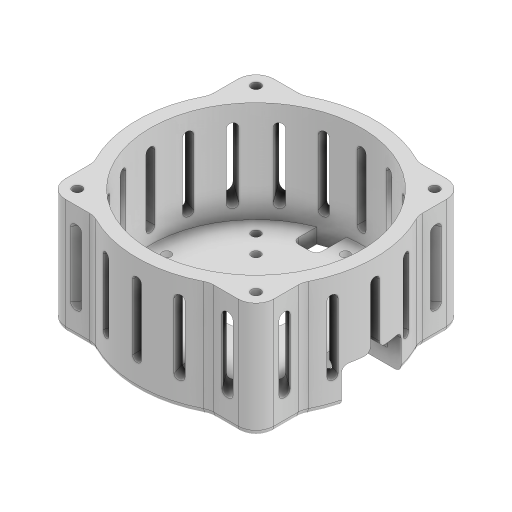
# Autodesk Inventor part: casing
Saved by Autodesk Inventor 2024.3 (Build 283343000, 343)
## iProperties
Created: 2025-08-30
Part Number: casing
Material: Generic
Document SubType Name: Modeling
Designer: danie
Density: 1 g/cm^3
Appearance: Default
Author: danie
Autodesk Inventor part; units mm, degrees
ref_plane "YZ Plane" through (0, 0, 0) normal (1, 0, 0) x (0, 1, 0)
ref_plane "XZ Plane" through (0, 0, 0) normal (0, 1, 0) x (-1, 0, 0)
ref_plane "XY Plane" through (0, 0, 0) normal (0, 0, 1) x (1, 0, 0)
sketch "Sketch1" plane through (0, 0, 0) normal (0, 1, 0) x (-1, 0, 0)
  circle A0 centre (0, 0) radius 34.5
  line L0 (-15, 15) -> (15, 15)
  line L1 (15, 15) -> (15, -15)
  line L2 (15, -15) -> (-15, -15)
  line L3 (-15, -15) -> (-15, 15)
  line L4 (-15, 15) -> (15, -15) construction
  line L5 (15, 15) -> (-15, -15) construction
  circle A1 centre (0, 0) radius 40
  circle A2 centre (0, 0) radius 35.5
  line L6 (-35, 35) -> (35, 35)
  line L7 (35, 35) -> (35, -35)
  line L8 (35, -35) -> (-35, -35)
  line L9 (-35, -35) -> (-35, 35)
  line L10 (-35, 35) -> (35, -35) construction
  line L11 (35, 35) -> (-35, -35) construction
  circle A3 centre (15, 15) radius 1.5
  circle A4 centre (15, -15) radius 1.5
  circle A5 centre (-15, -15) radius 1.5
  circle A6 centre (-15, 15) radius 1.5
  line L12 (21, 21) -> (-21, 21)
  line L13 (-21, 21) -> (-21, -21)
  line L14 (-21, -21) -> (21, -21)
  line L15 (21, -21) -> (21, 21)
  line L16 (21, 21) -> (-21, -21) construction
  line L17 (-21, 21) -> (21, -21) construction
  circle A7 centre (0, 0) radius 10
  circle A8 centre (21, 21) radius 1.5
  circle A9 centre (21, -21) radius 1.5
  circle A10 centre (-21, 21) radius 1.5
  circle A11 centre (-21, -21) radius 1.5
  line L18 (0, 0) -> (30, 0)
  circle A12 centre (30, 0) radius 1.5
  circle A13 centre (0, 30) radius 1.5
  circle A14 centre (-30, 0) radius 1.5
  circle A15 centre (0, -30) radius 1.5
  line L19 (-45.5, 10) -> (-27.5, 10)
  line L20 (-25.5, 8) -> (-25.5, -8)
  line L21 (-27.5, -10) -> (-45.5, -10)
  line L22 (-45.5, -10) -> (-45.5, 10)
  line L23 (-45.5, 10) -> (-25.5, -10) construction
  line L24 (-25.5, 10) -> (-45.5, -10) construction
  arc A16 (-25.5, 8) -> (-27.5, 10) centre (-27.5, 8) ccw
  arc A17 (-27.5, -10) -> (-25.5, -8) centre (-27.5, -8) ccw
  line L25 (0, 35) -> (0, -35)
  line L26 (35, 35) -> (0, 35)
  line L27 (17.5, 35) -> (17.5, -35)
  line L28 (17.5, 35) -> (0, 35)
  line L29 (8.75, 35) -> (8.75, -35)
  line L30 (4.75, 45) -> (12.75, 45)
  line L31 (12.75, 45) -> (12.75, 27)
  line L32 (10.75, 25) -> (6.75, 25)
  line L33 (4.75, 27) -> (4.75, 45)
  line L34 (4.75, 45) -> (12.75, 25) construction
  line L35 (12.75, 45) -> (4.75, 25) construction
  arc A18 (10.75, 25) -> (12.75, 27) centre (10.75, 27) ccw
  arc A19 (4.75, 27) -> (6.75, 25) centre (6.75, 27) ccw
  line L36 (4.75, -45) -> (12.75, -45)
  line L37 (12.75, -45) -> (12.75, -27)
  line L38 (10.75, -25) -> (6.75, -25)
  line L39 (4.75, -27) -> (4.75, -45)
  arc A20 (12.75, -27) -> (10.75, -25) centre (10.75, -27) ccw
  arc A21 (6.75, -25) -> (4.75, -27) centre (6.75, -27) ccw
  line L40 (-4.75, 45) -> (-12.75, 45)
  line L41 (-12.75, 45) -> (-12.75, 27)
  line L42 (-10.75, 25) -> (-6.75, 25)
  line L43 (-4.75, 27) -> (-4.75, 45)
  arc A22 (-12.75, 27) -> (-10.75, 25) centre (-10.75, 27) ccw
  arc A23 (-6.75, 25) -> (-4.75, 27) centre (-6.75, 27) ccw
  line L44 (-12.75, -45) -> (-12.75, -27)
  arc A24 (-10.75, -25) -> (-12.75, -27) centre (-10.75, -27) ccw
  line L45 (-10.75, -25) -> (-6.75, -25)
  arc A25 (-4.75, -27) -> (-6.75, -25) centre (-6.75, -27) ccw
  line L46 (-4.75, -27) -> (-4.75, -45)
  line L47 (-4.75, -45) -> (-12.75, -45)
  point P0 (19.3649, 35)
  point P1 (-19.3649, 35)
  point P2 (-35, 19.3649)
  point P3 (-35, -19.3649)
  point P4 (-19.3649, -35)
  point P5 (19.3649, -35)
  point P6 (35, -19.3649)
  point P7 (35, 19.3649)
  point P8 (-5.9372, -35)
  point P9 (5.9372, -35)
  point P10 (5.9372, 35)
  point P11 (-5.9372, 35)
  point P12 (-35.5, 0)
  point P13 (12.75, 33.1314)
  point P14 (4.75, 35.1808)
  point P15 (-4.75, 35.1808)
  point P16 (-12.75, 33.1314)
  point P17 (-34.0624, 10)
  point P18 (-34.0624, -10)
  point P19 (-12.75, -33.1314)
  point P20 (-4.75, -35.1808)
  point P21 (4.75, -35.1808)
  point P22 (12.75, -33.1314)
  dimension "d30" = 71
  dimension "d0" = 69
  dimension "d1" = 30
  dimension "d2" = 30
  dimension "d3" = 80
  dimension "d4" = 70
  dimension "d5" = 70
  dimension "d6" = 3
  dimension "d7" = 3
  dimension "d8" = 3
  dimension "d9" = 3
  dimension "d10" = 20
  dimension "d11" = 3
  dimension "d12" = 42
  dimension "d15" = 42
  dimension "d18" = 42
  dimension "d25" = 3
  dimension "d28" = 360
  dimension "d31" = 20
  dimension "d32" = 20
  dimension "d33" = 2
  dimension "d34" = 8
  dimension "d35" = 20
  dimension "d36" = 2
  constraints: 96 end point, 25 centre point, 24 symmetric about line, 20 point on circle, 14 midpoint, 11 point on line, 10 coincident, 10 parallel, 8 tangent, 7 horizontal, 7 perpendicular, 2 collinear, 2 equal radius, 1 vertical, 24 other
  measures "d0" diameter of A0
  measures "d1" distance between parallel lines of L2 L0
  measures "d2" distance between parallel lines of L3 L1
  measures "d3" diameter of A1
  measures "d4" distance between parallel lines of L8 L6
  measures "d5" distance between parallel lines of L9 L7
  measures "d6" diameter of A3
  measures "d7" diameter of A4
  measures "d8" diameter of A5
  measures "d9" diameter of A6
  measures "d10" diameter of A7
  measures "d11" diameter of A8
  measures "d12" distance between parallel lines of L14 L12
  measures "d15" distance of A8.centre A9.centre
  measures "d18" distance of A8.centre A10.centre
  measures "d25" diameter of A12
  measures "d31" distance between parallel lines of L21 L19
  measures "d32" distance between parallel lines of L22 L20
  measures "d33" radius of A16
  measures "d34" distance between parallel lines of L33 L31
  measures "d35" distance between parallel lines of L30 L32
  measures "d36" radius of A18
extrude "Extrusion1" add sketch "Sketch1" along normal blind 39 contours L27 L6 A1 L7 A2 | A2 L31 L6 L27 | L27 L8 L37 A2 | A2 L7 A1 L8 L27 | A2 L29 L6 L31 | L7 A1 A2 | L6 L31 A1 | L37 L8 L29 A2 | L8 A1 L37 | A2 L6 L29 | L6 A2 L33 A1 L31 | A1 L6 L7 | L29 L8 A2 | L37 A1 L39 A2 L8 | L7 L8 A1 | A2 L43 A1 L33 | L39 A1 L46 A2 | A2 L6 L41 A1 L43 | L46 A1 L44 L8 A2 | L41 L6 A2 | A2 L19 L9 A1 L6 L41 | L41 L6 A1 | L44 L8 A1 L9 L21 A2 | A2 L8 L44 | A1 L8 L44 | A2 L9 L19 | A1 L9 L6 | L21 L9 A2 | L8 L9 A1 | A2 L9 L21 A1 L19 | L19 A1 L9 | L9 A1 L21
extrude "Extrusion2" add sketch "Sketch1" along normal blind 5 contours A0 L27 L14 A9 L15 A8 L12 | A0 L27 A2 L7 | L27 L12 L29 L32 A18 L31 A0 | A0 L31 A2 L27 | L27 A2 L37 A0 | A0 L37 A20 L38 L29 L14 L27 | L27 L18 L1 A3 L0 L29 L12 | L12 A8 L15 L18 L27 | L27 L18 L15 A9 L14 | L14 L29 L2 A4 L1 L18 L27 | A2 L7 | L29 L0 L25 L12 | L12 L25 A13 A0 L33 A19 L32 L29 | L29 L38 A21 L39 A0 L25 A15 L14 | L14 L25 L2 L29 | A0 L25 L6 L33 | L25 L0 A6 L3 A5 L2 L14 A11 L13 A10 L12 | L12 A10 L13 A11 L14 L25 A15 A0 L46 A25 L45 A24 L44 L21 A17 L20 A16 L19 L41 A22 L42 A23 L43 A13 | L29 A7 L25 L0 | L0 A3 L1 L18 A7 L29 | L1 A4 L2 L29 A7 L18 | L39 L8 L25 A0 | L2 L25 A7 L29 | A0 L43 L6 L25 | L6 L43 A2 L33 | L25 A7 L2 A5 L3 A6 L0 | L25 L8 L46 A0 | L39 A2 L46 L8 | A0 L19 A2 L41 | L44 A2 L21 A0
sketch "Sketch3" plane through (0, 0, 0) normal (0, -1, 0) x (1, 0, 0)
  arc A0 (-4.75, 35.1808) -> (-12.75, 33.1314) centre (0, 0) ccw projected
  line L0 (-4.75, 27) -> (-4.75, 35.1808) projected
  arc A1 (-6.75, 25) -> (-4.75, 27) centre (-6.75, 27) ccw projected
  line L1 (-10.75, 25) -> (-6.75, 25) projected
  arc A2 (-12.75, 27) -> (-10.75, 25) centre (-10.75, 27) ccw projected
  line L2 (-12.75, 33.1314) -> (-12.75, 27) projected
  line L3 (-12.75, -27) -> (-12.75, -33.1314) projected
  arc A3 (-10.75, -25) -> (-12.75, -27) centre (-10.75, -27) ccw projected
  line L4 (-6.75, -25) -> (-10.75, -25) projected
  arc A4 (-4.75, -27) -> (-6.75, -25) centre (-6.75, -27) ccw projected
  line L5 (-4.75, -35.1808) -> (-4.75, -27) projected
  arc A5 (-12.75, -33.1314) -> (-4.75, -35.1808) centre (0, 0) ccw projected
  line L6 (4.75, -27) -> (4.75, -35.1808) projected
  arc A6 (6.75, -25) -> (4.75, -27) centre (6.75, -27) ccw projected
  line L7 (10.75, -25) -> (6.75, -25) projected
  arc A7 (12.75, -27) -> (10.75, -25) centre (10.75, -27) ccw projected
  line L8 (12.75, -33.1314) -> (12.75, -27) projected
  arc A8 (4.75, -35.1808) -> (12.75, -33.1314) centre (0, 0) ccw projected
  line L9 (27.5, -10) -> (34.0624, -10) projected
  arc A9 (25.5, -8) -> (27.5, -10) centre (27.5, -8) ccw projected
  line L10 (25.5, 8) -> (25.5, -8) projected
  arc A10 (27.5, 10) -> (25.5, 8) centre (27.5, 8) ccw projected
  line L11 (34.0624, 10) -> (27.5, 10) projected
  arc A11 (34.0624, -10) -> (34.0624, 10) centre (0, 0) ccw projected
  circle A12 centre (-15, -15) radius 1.5 projected
  circle A13 centre (-21, 21) radius 1.5 projected
  circle A14 centre (0, 30) radius 1.5 projected
  circle A15 centre (21, -21) radius 1.5 projected
  circle A16 centre (0, -30) radius 1.5 projected
  circle A17 centre (21, 21) radius 1.5 projected
  circle A18 centre (-15, 15) radius 1.5 projected
  circle A19 centre (0, 0) radius 10 projected
  circle A20 centre (15, -15) radius 1.5 projected
  circle A21 centre (15, 15) radius 1.5 projected
  circle A22 centre (-30, 0) radius 1.5 projected
  circle A23 centre (-21, -21) radius 1.5 projected
  line L12 (19.3649, 35) -> (35, 35) projected
  arc A24 (19.3649, 35) -> (-19.3649, 35) centre (0, 0) ccw projected
  line L13 (-35, 35) -> (-19.3649, 35) projected
  line L14 (-35, 19.3649) -> (-35, 35) projected
  arc A25 (-35, 19.3649) -> (-35, -19.3649) centre (0, 0) ccw projected
  line L15 (-35, -35) -> (-35, -19.3649) projected
  line L16 (-19.3649, -35) -> (-35, -35) projected
  arc A26 (-19.3649, -35) -> (19.3649, -35) centre (0, 0) ccw projected
  line L17 (35, -35) -> (19.3649, -35) projected
  line L18 (35, -19.3649) -> (35, -35) projected
  arc A27 (35, -19.3649) -> (35, 19.3649) centre (0, 0) ccw projected
  line L19 (35, 35) -> (35, 19.3649) projected
  line L20 (12.75, 27) -> (12.75, 33.1314) projected
  arc A28 (10.75, 25) -> (12.75, 27) centre (10.75, 27) ccw projected
  line L21 (6.75, 25) -> (10.75, 25) projected
  arc A29 (4.75, 27) -> (6.75, 25) centre (6.75, 27) ccw projected
  line L22 (4.75, 35.1808) -> (4.75, 27) projected
  arc A30 (12.75, 33.1314) -> (4.75, 35.1808) centre (0, 0) ccw projected
  line L23 (34.0624, 10) -> (38.7298, 10)
  line L24 (34.0624, -10) -> (38.7298, -10)
  constraints: 4 end point, 2 point on circle, 1 horizontal, 1 parallel
extrude "Extrusion3" cut sketch "Sketch3" against normal blind 12 contours A11 L23 A27 L24
fillet "Fillet1" radius 2 2 edges at (36.3961, 12, 10) (36.3961, 12, -10)
ref_plane "Work Plane1" through (-35, 0, 0) normal (0, 0, 1) x (1, 0, 0)
sketch "Sketch4" plane through (-35, 0, 0) normal (0, 0, 1) x (1, 0, 0)
  line L0 (22.25, 5) -> (24.25, 5) projected
  line L1 (24.25, 5) -> (28.25, 5) projected
  line L2 (28.25, 5) -> (30.25, 5) projected
  line L3 (30.25, 5) -> (30.25, 5) projected
  line L4 (39.75, 5) -> (41.75, 5) projected
  line L5 (41.75, 5) -> (45.75, 5) projected
  line L6 (45.75, 5) -> (47.75, 5) projected
  line L7 (69.0624, 5) -> (47.75, 5) projected
  line L8 (69.0624, 5) -> (62.5, 5) projected
  line L9 (62.5, 5) -> (60.5, 5) projected
  line L10 (60.5, 5) -> (62.5, 5) projected
  line L11 (62.5, 5) -> (69.0624, 5) projected
  line L12 (47.75, 5) -> (69.0624, 5) projected
  line L13 (47.75, 5) -> (45.75, 5) projected
  line L14 (45.75, 5) -> (41.75, 5) projected
  line L15 (41.75, 5) -> (39.75, 5) projected
  line L16 (30.25, 5) -> (39.75, 5) projected
  line L17 (30.25, 5) -> (28.25, 5) projected
  line L18 (28.25, 5) -> (24.25, 5) projected
  line L19 (24.25, 5) -> (22.25, 5) projected
  line L20 (22.25, 5) -> (22.25, 5) projected
  line L21 (12.5, 5) -> (15.5, 5) projected
  line L22 (3.5, 5) -> (6.5, 5) projected
  line L23 (48.5, 5) -> (51.5, 5) projected
  line L24 (48.5, 5) -> (51.5, 5) projected
  line L25 (25, 5) -> (45, 5) projected
  line L26 (18.5, 5) -> (21.5, 5) projected
  line L27 (54.5, 5) -> (57.5, 5) projected
  line L28 (33.5, 5) -> (36.5, 5) projected
  line L29 (54.5, 5) -> (57.5, 5) projected
  line L30 (33.5, 5) -> (36.5, 5) projected
  line L31 (12.5, 5) -> (15.5, 5) projected
  line L32 (18.5, 5) -> (21.5, 5) projected
  line L33 (30.25, 5) -> (30.25, 5) projected
  line L34 (15.6351, 0) -> (54.3649, 0) projected
  line L35 (54.3649, 0) -> (54.3649, 39) projected
  line L36 (15.6351, 39) -> (54.3649, 39) projected
  line L37 (15.6351, 0) -> (15.6351, 39) projected
  line L38 (15.6351, 39) -> (54.3649, 39)
  line L39 (54.3649, 39) -> (54.3649, 0)
  line L40 (54.3649, 0) -> (15.6351, 0)
  line L41 (15.6351, 0) -> (15.6351, 39)
  line L42 (35, 39) -> (35, 0)
  line L43 (35, 32) -> (35, 10) construction
  line L44 (33.5, 32) -> (33.5, 10)
  line L45 (36.5, 10) -> (36.5, 32)
  arc A0 (36.5, 32) -> (33.5, 32) centre (35, 32) ccw
  arc A1 (33.5, 10) -> (36.5, 10) centre (35, 10) ccw
  point P0 (35, 21)
  point P1 (35, 33.5)
  point P2 (35, 8.5)
  dimension "d40" = 3
  dimension "d41" = 18
  dimension "d42" = 25
  constraints: 18 end point, 6 point on circle, 4 tangent, 3 parallel, 2 centre point, 2 midpoint, 2 point on line, 1 horizontal, 1 perpendicular, 1 vertical, 1 other
  measures "d40" distance between parallel lines of L45 L44
  measures "d41" distance from line of L38 point (35, 21)
  measures "d42" distance of point (35, 33.5) point (35, 8.5)
extrude "Extrusion4" cut sketch "Sketch4" along normal blind 70 contours A1 L44 A0 L42 | L42 A0 L45 A1
pattern_circular "Circular Pattern2" count 20 over 360 about axis through (0, 0, 0) along (0, 1, 0) of "Extrusion4"
sketch "Sketch5" plane through (0, 0, 0) normal (0, -1, 0) x (1, 0, 0)
  line L0 (30, -30) -> (-30, -30)
  line L1 (-30, -30) -> (-30, 30)
  line L2 (-30, 30) -> (30, 30)
  line L3 (30, 30) -> (30, -30)
  line L4 (30, -30) -> (-30, 30) construction
  line L5 (-30, -30) -> (30, 30) construction
  point P0 (0, 0)
  dimension "d53" = 60
  dimension "d54" = 60
  constraints: 12 end point, 2 midpoint, 2 parallel, 1 horizontal, 1 perpendicular
  measures "d53" distance between parallel lines of L2 L0
  measures "d54" distance between parallel lines of L3 L1
hole "Hole1" at (30, 0, -30) at (30, 0, 30) at (-30, 0, 30) at (-30, 0, -30) direction (0, 1, 0) diameter 3.175 depth 50 tip angle 118 counterbore diameter 6.3 counterbore depth 20
fillet "Fillet4" radius 6 12 edges at (19.3649, 19.5, 35) (-19.3649, 19.5, 35) (-35, 19.5, 19.3649) (-35, 19.5, -19.3649) (-19.3649, 19.5, -35) (19.3649, 19.5, -35) (35, 19.5, -19.3649) (35, 19.5, 19.3649) (35, 19.5, -35) (-35, 19.5, -35) (35, 19.5, 35) (-35, 19.5, 35)
fillet "Fillet5" radius 2 25 edges at (33.2426, 0, -33.2426) (24.9283, 0, -35) (19.4579, 0, -35.1653) (0, 0, -40) (-19.4579, 0, -35.1653) (-24.9283, 0, -35) (-33.2426, 0, -33.2426) (-35, 0, -24.9283) (-35.1653, 0, -19.4579) (-40, 0, 0) (-35.1653, 0, 19.4579) (-35, 0, 24.9283) (-33.2426, 0, 33.2426) (-24.9283, 0, 35) (-19.4579, 0, 35.1653) (0, 0, 40) (19.4579, 0, 35.1653) (24.9283, 0, 35) (33.2426, 0, 33.2426) (35, 0, 24.9283) (35.1653, 0, 19.4579) (37.4128, 0, 14.152) (35.1653, 0, -19.4579) (37.4128, 0, -14.152) (35, 0, -24.9283)
fillet "Fillet6" radius 2 2 edges at (37.7201, 12, 1.5) (37.7201, 12, -1.5)
body "Solid1"
